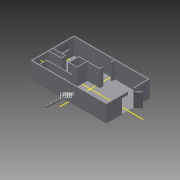
# Autodesk Inventor part: West_Structure_Hose_Test_2nd_Floor
Saved by Autodesk Inventor 2013 SP2 (Build 170200200, 200)
## iProperties
Created: 2013-07-10
Part Number: West_Structure_Hose_Test_2nd_Floor
Material: Generic
Document SubType Name: Modeling
Designer: jmw3
Density: 1 g/cm^3
Author: jmw3
Autodesk Inventor part; units mm, degrees
ref_plane "YZ Plane" through (0, 0, 0) normal (1, 0, 0) x (0, 1, 0)
ref_plane "XZ Plane" through (0, 0, 0) normal (0, 1, 0) x (-1, 0, 0)
ref_plane "XY Plane" through (0, 0, 0) normal (0, 0, 1) x (1, 0, 0)
sketch "Sketch1" plane through (0, 0, 0) normal (0, 0, 1) x (1, 0, 0)
  line L0 (-5588, 3200.4) -> (5588, 3200.4)
  line L1 (5588, -3200.4) -> (-5588, -3200.4)
  line L2 (-3958.3754, 3048) -> (-719.8754, 3048)
  line L3 (5435.6, 914.4) -> (5588, 914.4)
  line L4 (5588, -914.4) -> (5435.6, -914.4)
  line L5 (-4072.6754, 3048) -> (-605.5754, 3048)
  line L6 (5588, 3200.4) -> (5588, 914.4)
  line L7 (5588, -914.4) -> (5588, -3200.4)
  line L8 (5435.6, 3048) -> (5435.6, 914.4)
  line L9 (5435.6, -914.4) -> (5435.6, -3048)
  line L10 (-5588, 894.5564) -> (-5588, 3200.4)
  line L11 (-5435.6, 76.2) -> (-5435.6, 3048)
  line L12 (0, -4480.56) -> (0, 4480.56) projected
  line L13 (-7823.2, 0) -> (7823.2, 0) projected
  line L14 (-863.6, -3048) -> (-863.6, -2006.6)
  line L15 (-863.6, -2006.6) -> (-4381.5, -2006.6)
  line L16 (-4495.8, -2006.6) -> (-4495.8, -3048)
  line L17 (-5435.6, 76.2) -> (-3581.4, 76.2)
  line L18 (-3581.4, 76.2) -> (-3581.4, -685.8)
  line L19 (-3581.4, -685.8) -> (-5435.6, -685.8)
  line L20 (-5435.6, -571.5) -> (-5435.6, -38.1)
  line L21 (-5435.6, -38.1) -> (-3695.7, -38.1)
  line L22 (-3695.7, -38.1) -> (-3695.7, -571.5)
  line L23 (-3695.7, -571.5) -> (-5435.6, -571.5)
  line L24 (-5435.6, -571.5) -> (-5435.6, -38.1)
  line L25 (-5588, -965.2) -> (-5435.6, -965.2)
  line L26 (-5435.6, -1879.6) -> (-5588, -1879.6)
  line L27 (-5435.6, -3048) -> (-5435.6, -1879.6)
  line L28 (-5588, -3200.4) -> (-5588, -1879.6)
  line L29 (-5588, -965.2) -> (-5588, 914.4)
  line L30 (-2590.8, 914.4) -> (-1377.4097, 914.4)
  line L31 (-1244.6, 800.1) -> (-1244.6, -685.8)
  line L32 (-1244.6, -685.8) -> (-2590.8, -685.8)
  line L33 (-2590.8, -685.8) -> (-2590.8, 914.4)
  line L34 (-1377.4097, 914.4) -> (508, 914.4)
  line L35 (622.3, 952.5) -> (622.3, 800.1)
  line L36 (622.3, 800.1) -> (-1244.6, 800.1)
  line L37 (508, 914.4) -> (508, 1314.45)
  line L38 (508, 1314.45) -> (622.3, 1314.45)
  line L39 (622.3, 1314.45) -> (622.3, 800.1)
  line L40 (622.3, 3048) -> (622.3, 2533.65)
  line L41 (622.3, 2533.65) -> (508, 2533.65)
  line L42 (508, 2533.65) -> (508, 3048)
  line L43 (-2476.5, 800.1) -> (-1358.9, 800.1)
  line L44 (-1358.9, 800.1) -> (-1358.9, -571.5)
  line L45 (-1358.9, -571.5) -> (-2476.5, -571.5)
  line L46 (-2476.5, -571.5) -> (-2476.5, 800.1)
  line L47 (-749.3, -3048) -> (-749.3, -1892.3)
  line L48 (-749.3, -1892.3) -> (-4495.8, -1892.3)
  line L49 (-4495.8, -1892.3) -> (-4495.8, -2006.6)
  line L50 (-5435.6, 3048) -> (508, 3048)
  line L51 (622.3, 3048) -> (5435.6, 3048)
  line L52 (-4381.5, -2006.6) -> (-4381.5, -3048)
  line L53 (-863.6, -2006.6) -> (-1060.3581, -2006.6)
  line L54 (-5435.6, -965.2) -> (-5435.6, -685.8)
  line L55 (-5435.6, -571.5) -> (-5435.6, -38.1)
  line L56 (-4495.8, -3048) -> (-5435.6, -3048)
  line L57 (5435.6, -3048) -> (-749.3, -3048)
  line L58 (-863.6, -3048) -> (-4381.5, -3048)
  line L59 (880.3246, -3048) -> (-749.3, -3048)
  line L60 (-5435.6, -38.1) -> (-5435.6, -571.5)
  line L61 (-5435.6, -685.8) -> (-5435.6, -965.2)
  line L62 (-5435.6, -685.8) -> (-3581.4, -685.8)
  line L63 (-5435.6, 76.2) -> (-3581.4, 76.2)
  line L64 (-5435.6, 76.2) -> (-5435.6, 3048)
  line L65 (-5435.6, -685.8) -> (-5435.6, -965.2)
  line L66 (-5435.6, -965.2) -> (-5588, -965.2)
  line L67 (-5588, -965.2) -> (-5588, 3200.4)
  line L68 (-5435.6, 3048) -> (-5435.6, 76.2)
  line L69 (-5435.6, 76.2) -> (-3581.4, 76.2)
  line L70 (-3581.4, 76.2) -> (-3581.4, -685.8)
  line L71 (-3581.4, -685.8) -> (-5435.6, -685.8)
  line L72 (-5435.6, -571.5) -> (-3695.7, -571.5)
  line L73 (-3695.7, -571.5) -> (-3695.7, -38.1)
  line L74 (-3695.7, -38.1) -> (-5435.6, -38.1)
  line L75 (-5435.6, -38.1) -> (-5435.6, -571.5)
  dimension "d14" = 1828.8
  dimension "d90" = 6299.2
  dimension "d94" = 114.3
  dimension "d95" = 114.3
  dimension "d96" = 114.3
  dimension "d99" = 914.4
  dimension "d100" = 152.4
  dimension "d102" = 939.8
  dimension "d104" = 990.6
  dimension "d105" = 114.3
  dimension "d106" = 114.3
  dimension "d107" = 114.3
  dimension "d108" = 114.3
  dimension "d109" = 114.3
  dimension "d110" = 6680.2
  dimension "d112" = 1219.2
  dimension "d120" = 152.4
  dimension "d122" = 2971.8
  dimension "d123" = 2286
  dimension "d124" = 5943.6
  dimension "d125" = 114.3
  dimension "d127" = 114.3
  dimension "d128" = 6400.8
  dimension "d129" = 152.4
  dimension "d130" = 1168.4
  dimension "d131" = 1041.4
  dimension "d132" = 114.3
  dimension "d133" = 1854.2
  dimension "d134" = 2362.2
  dimension "d135" = 10871.2
  dimension "d236" = 2133.6
  dimension "d237" = 514.35
  dimension "d238" = 114.3
  constraints: 148 end point, 38 parallel, 28 perpendicular, 26 collinear, 12 horizontal, 3 point on line, 3 other
  measures "d14" distance between parallel lines of L4 L3
  measures "d90" distance between parallel lines of L9 L14
  measures "d94" distance between parallel lines of L19 L23
  measures "d95" distance between parallel lines of L18 L22
  measures "d96" distance between parallel lines of L17 L21
  measures "d99" distance between parallel lines of L25 L26
  measures "d100" distance between parallel lines of L10 L11
  measures "d102" distance between parallel lines of L27 L16
  measures "d104" distance between parallel lines of L18 L33
  measures "d105" distance between parallel lines of L33 L46
  measures "d106" distance between parallel lines of L31 L44
  measures "d107" distance between parallel lines of L32 L45
  measures "d108" distance between parallel lines of L30 L43
  measures "d109" distance between parallel lines of L39 L37
  measures "d110" distance between parallel lines of L8 L31
  measures "d112" distance from line of L38.end L41
  measures "d120" distance between parallel lines of L50 L0
  measures "d122" distance between parallel lines of L50 L17
  measures "d123" distance between parallel lines of L1 L4
  measures "d124" distance between parallel lines of L11 L37
  measures "d125" distance between parallel lines of L16 L52
  measures "d127" distance between parallel lines of L14 L47
  measures "d128" distance between parallel lines of L1 L0
  measures "d129" distance between parallel lines of L1 L57
  measures "d130" distance between parallel lines of L56 L26
  measures "d131" distance between parallel lines of L58 L15
  measures "d132" distance between parallel lines of L15 L48
  measures "d133" distance between parallel lines of L54 L18
  measures "d134" distance between parallel lines of L56 L19
  measures "d135" distance between parallel lines of L9 L27
  measures "d236" distance between parallel lines of L50 L30
  measures "d237" distance between parallel lines of L36 L38
  measures "d238" distance of L40.end L41.end
extrude "Extrusion7" add sketch "Sketch1" along normal blind 2463.8 contours L57 L9 L4 L7 L1 L12 | L12 L1 L28 L26 L27 L56 L16 L49 L48 L47 L57 | L0 L12 L50 L5 L2 L11 L17 L18 L13 L29 L10 | L0 L6 L3 L8 L51 L40 L41 L42 L50 L12 | L34 L37 L38 L39 L35 L36 L12 | L12 L36 L31 L13 L44 L43 L46 L33 L30 L34 | L13 L18 L19 L54 L25 L29 | L13 L46 L45 L44 L31 L32 L33
sketch "Sketch4" plane through (0, 0, 0) normal (0, 0, -1) x (-1, 0, 0)
  line L0 (4381.5, -3048) -> (863.6, -3048) projected
  line L1 (863.6, -3048) -> (863.6, -2006.6) projected
  line L2 (863.6, -2006.6) -> (4381.5, -2006.6) projected
  line L3 (4381.5, -2006.6) -> (4381.5, -3048) projected
  line L4 (-5435.6, -3048) -> (749.3, -3048) projected
  line L5 (-5435.6, -914.4) -> (-5435.6, -3048) projected
  line L6 (-5588, -914.4) -> (-5435.6, -914.4) projected
  line L7 (-5588, -3200.4) -> (-5588, -914.4) projected
  line L8 (5588, -3200.4) -> (-5588, -3200.4) projected
  line L9 (5588, -1879.6) -> (5588, -3200.4) projected
  line L10 (5435.6, -1879.6) -> (5588, -1879.6) projected
  line L11 (5435.6, -3048) -> (5435.6, -1879.6) projected
  line L12 (4495.8, -3048) -> (5435.6, -3048) projected
  line L13 (4495.8, -1892.3) -> (4495.8, -3048) projected
  line L14 (749.3, -1892.3) -> (4495.8, -1892.3) projected
  line L15 (749.3, -3048) -> (749.3, -1892.3) projected
  line L16 (3695.7, -571.5) -> (3695.7, -38.1) projected
  line L17 (3695.7, -38.1) -> (5435.6, -38.1) projected
  line L18 (5435.6, -38.1) -> (5435.6, -571.5) projected
  line L19 (5435.6, -571.5) -> (3695.7, -571.5) projected
  line L20 (5435.6, 3048) -> (-508, 3048) projected
  line L21 (5435.6, 76.2) -> (5435.6, 3048) projected
  line L22 (3581.4, 76.2) -> (5435.6, 76.2) projected
  line L23 (3581.4, -685.8) -> (3581.4, 76.2) projected
  line L24 (5435.6, -685.8) -> (3581.4, -685.8) projected
  line L25 (5435.6, -965.2) -> (5435.6, -685.8) projected
  line L26 (5588, -965.2) -> (5435.6, -965.2) projected
  line L27 (5588, 3200.4) -> (5588, -965.2) projected
  line L28 (-5588, 3200.4) -> (5588, 3200.4) projected
  line L29 (-5588, 914.4) -> (-5588, 3200.4) projected
  line L30 (-5435.6, 914.4) -> (-5588, 914.4) projected
  line L31 (-5435.6, 3048) -> (-5435.6, 914.4) projected
  line L32 (-622.3, 3048) -> (-5435.6, 3048) projected
  line L33 (-622.3, 2533.65) -> (-622.3, 3048) projected
  line L34 (-508, 2533.65) -> (-622.3, 2533.65) projected
  line L35 (-508, 3048) -> (-508, 2533.65) projected
  line L36 (1358.9, -571.5) -> (1358.9, 800.1) projected
  line L37 (1358.9, 800.1) -> (2476.5, 800.1) projected
  line L38 (2476.5, 800.1) -> (2476.5, -571.5) projected
  line L39 (2476.5, -571.5) -> (1358.9, -571.5) projected
  line L40 (2590.8, 914.4) -> (-508, 914.4) projected
  line L41 (-508, 914.4) -> (-508, 1314.45) projected
  line L42 (-508, 1314.45) -> (-622.3, 1314.45) projected
  line L43 (-622.3, 1314.45) -> (-622.3, 800.1) projected
  line L44 (-622.3, 800.1) -> (1244.6, 800.1) projected
  line L45 (1244.6, 800.1) -> (1244.6, -685.8) projected
  line L46 (1244.6, -685.8) -> (2590.8, -685.8) projected
  line L47 (2590.8, -685.8) -> (2590.8, 914.4) projected
  line L48 (-5588, 3200.4) -> (5588, 3200.4)
  line L49 (5588, 3200.4) -> (5588, -2006.6)
  line L50 (5588, -2006.6) -> (-5588, -2006.6)
  line L51 (-5588, -2006.6) -> (-5588, 3200.4)
  line L52 (-5588, -2006.6) -> (863.6, -2006.6)
  line L53 (863.6, -2006.6) -> (863.6, -3200.4)
  line L54 (863.6, -3200.4) -> (-5588, -3200.4)
  line L55 (-5588, -3200.4) -> (-5588, -2006.6)
  line L56 (4381.5, -2006.6) -> (5588, -2006.6)
  line L57 (5588, -2006.6) -> (5588, -3200.4)
  line L58 (5588, -3200.4) -> (4381.5, -3200.4)
  line L59 (4381.5, -3200.4) -> (4381.5, -2006.6)
  line L60 (4381.5, -3048) -> (863.6, -3048)
  line L61 (863.6, -3048) -> (863.6, -3200.4)
  line L62 (863.6, -3200.4) -> (4381.5, -3200.4)
  line L63 (4381.5, -3200.4) -> (4381.5, -3048)
  line L64 (863.6, -3200.4) -> (4381.5, -3200.4)
  line L65 (4381.5, -3200.4) -> (4381.5, -2895.6)
  line L66 (4381.5, -2895.6) -> (863.6, -2895.6)
  line L67 (863.6, -2895.6) -> (863.6, -3200.4)
  point P0 (0, 0)
  dimension "d192" = 889
  constraints: 40 end point, 10 parallel, 5 horizontal, 5 perpendicular, 3 point on line
  measures "d192" distance between parallel lines of L66 L2
extrude "Extrusion8" add sketch "Sketch4" against normal blind 25.4 contours L59 L8 L53 L0 | L3 L50 L13 L12 L11 L9 L8 L59 | L53 L8 L7 L50 L5 L4 L15 L1 | L2 L50 L15 L14 L13 | L50 L11 L12 L13 | L13 L14 L15 L50 L5 L6 L51 L30 L31 L32 L33 L34 L35 L20 L21 L22 L23 L24 L25 L26 L49 L10 L11 | L50 L11 L10 L9 | L15 L4 L5 L50 | L7 L6 L5 L50 | L26 L25 L24 L23 L22 L21 L20 L35 L34 L33 L32 L31 L30 L29 L28 L27 | L16 L17 L18 L19 | L36 L37 L38 L39 | L47 L46 L45 L44 L43 L42 L41 L40
sketch "Sketch5" plane through (-749.3, -3048, 2463.8) normal (1, 0, 0) x (0, 0, -1)
  line L0 (2438.4, 0) -> (2438.4, 1155.7) projected
  line L1 (2438.4, 1155.7) -> (0, 1155.7) projected
  line L2 (2438.4, 114.3) -> (406.4, 114.3)
  line L3 (406.4, 114.3) -> (406.4, 927.1)
  line L4 (406.4, 927.1) -> (2438.4, 927.1)
  line L5 (2438.4, 927.1) -> (2438.4, 114.3)
  line L6 (2438.4, 165.1) -> (457.2, 165.1)
  line L7 (457.2, 165.1) -> (457.2, 876.3)
  line L8 (457.2, 876.3) -> (2438.4, 876.3)
  line L9 (2438.4, 876.3) -> (2438.4, 165.1)
  point P0 (2463.8, 3048)
  dimension "d140" = 2032
  dimension "d142" = 228.6
  dimension "d143" = 812.8
  dimension "d144" = 1981.2
  dimension "d145" = 711.2
  dimension "d146" = 50.8
  constraints: 16 end point, 4 parallel, 2 horizontal, 2 perpendicular, 2 point on line
  measures "d140" distance between parallel lines of L5 L3
  measures "d142" distance between parallel lines of L1 L4
  measures "d143" distance between parallel lines of L4 L2
  measures "d144" distance between parallel lines of L9 L7
  measures "d145" distance between parallel lines of L6 L8
  measures "d146" distance between parallel lines of L2 L6
extrude "Extrusion9" cut sketch "Sketch5" against normal blind 50.8 contours L2 L3 L4 L0 L8 L7 L6
extrude "Extrusion10" cut sketch "Sketch5" against normal up to surface (114.3 mm away) contours L6 L7 L8 L0
sketch "Sketch6" plane through (0, 0, 2463.8) normal (0, 0, 1) x (1, 0, 0)
  line L0 (-3695.7, -38.1) -> (-3695.7, -571.5) projected
  line L1 (-3695.7, -571.5) -> (-5435.6, -571.5) projected
  line L2 (-5435.6, -571.5) -> (-5435.6, -38.1) projected
  line L3 (-5435.6, -38.1) -> (-3695.7, -38.1) projected
  line L4 (-5435.6, 3048) -> (508, 3048) projected
  line L5 (508, 3048) -> (508, 2533.65) projected
  line L6 (508, 2533.65) -> (622.3, 2533.65) projected
  line L7 (622.3, 2533.65) -> (622.3, 3048) projected
  line L8 (622.3, 3048) -> (5435.6, 3048) projected
  line L9 (5435.6, 3048) -> (5435.6, 914.4) projected
  line L10 (5435.6, 914.4) -> (5588, 914.4) projected
  line L11 (5588, 914.4) -> (5588, 3200.4) projected
  line L12 (5588, 3200.4) -> (-5588, 3200.4) projected
  line L13 (-5588, 3200.4) -> (-5588, -965.2) projected
  line L14 (-5588, -965.2) -> (-5435.6, -965.2) projected
  line L15 (-5435.6, -965.2) -> (-5435.6, -685.8) projected
  line L16 (-5435.6, -685.8) -> (-3581.4, -685.8) projected
  line L17 (-3581.4, -685.8) -> (-3581.4, 76.2) projected
  line L18 (-3581.4, 76.2) -> (-5435.6, 76.2) projected
  line L19 (-5435.6, 76.2) -> (-5435.6, 3048) projected
  line L20 (-1358.9, 800.1) -> (-1358.9, -571.5) projected
  line L21 (-1358.9, -571.5) -> (-2476.5, -571.5) projected
  line L22 (-2476.5, -571.5) -> (-2476.5, 800.1) projected
  line L23 (-2476.5, 800.1) -> (-1358.9, 800.1) projected
  line L24 (508, 914.4) -> (-2590.8, 914.4) projected
  line L25 (-2590.8, 914.4) -> (-2590.8, -685.8) projected
  line L26 (-2590.8, -685.8) -> (-1244.6, -685.8) projected
  line L27 (-1244.6, -685.8) -> (-1244.6, 800.1) projected
  line L28 (-1244.6, 800.1) -> (622.3, 800.1) projected
  line L29 (622.3, 800.1) -> (622.3, 1314.45) projected
  line L30 (622.3, 1314.45) -> (508, 1314.45) projected
  line L31 (508, 1314.45) -> (508, 914.4) projected
  line L32 (5435.6, 914.4) -> (5588, 914.4)
  line L33 (5588, 914.4) -> (5588, -914.4)
  line L34 (5588, -914.4) -> (5435.6, -914.4)
  line L35 (5435.6, -914.4) -> (5435.6, 914.4)
  line L36 (-5588, -965.2) -> (-5435.6, -965.2)
  line L37 (-5435.6, -965.2) -> (-5435.6, -1879.6)
  line L38 (-5435.6, -1879.6) -> (-5588, -1879.6)
  line L39 (-5588, -1879.6) -> (-5588, -965.2)
  point P0 (0, 0)
  constraints: 16 end point, 4 parallel, 2 horizontal, 2 perpendicular
extrude "Extrusion11" add sketch "Sketch6" against normal blind 406.4 contours L37 L38 L39 L14 | L10 L33 L34 L35
sketch "Sketch7" plane through (-5435.6, 76.2, 2463.8) normal (1, 0, 0) x (0, 0, -1)
  line L0 (2438.4, 0) -> (2438.4, 2971.8) projected
  line L1 (2438.4, 2971.8) -> (0, 2971.8) projected
  line L2 (431.8, 647.7) -> (1346.2, 647.7)
  line L3 (1346.2, 647.7) -> (1346.2, 2324.1)
  line L4 (1346.2, 2324.1) -> (431.8, 2324.1)
  line L5 (431.8, 2324.1) -> (431.8, 647.7)
  point P0 (2463.8, -76.2)
  dimension "d153" = 1676.4
  dimension "d155" = 914.4
  dimension "d156" = 1092.2
  dimension "d157" = 647.7
  constraints: 8 end point, 2 parallel, 1 horizontal, 1 perpendicular
  measures "d153" distance between parallel lines of L2 L4
  measures "d155" distance between parallel lines of L5 L3
  measures "d156" distance between parallel lines of L0 L3
  measures "d157" distance between parallel lines of L1 L4
extrude "Extrusion12" cut sketch "Sketch7" against normal up to surface (152.4 mm away)
sketch "Sketch9" plane through (-863.6, -3048, 2463.8) normal (-1, 0, 0) x (0, 0, 1)
  line L0 (-2463.8, 0) -> (-2438.4, 0)
  line L1 (-2438.4, 0) -> (-2438.4, 152.4)
  line L2 (-2438.4, 152.4) -> (-2463.8, 152.4)
  line L3 (-2463.8, 152.4) -> (-2463.8, 0)
  point P0 (-2463.8, 3048)
  dimension "d193" = 152.4
  constraints: 8 end point, 2 parallel, 1 horizontal, 1 perpendicular
  measures "d193" distance between parallel lines of L2 L0
extrude "Extrusion14" add sketch "Sketch9" along normal up to surface (3517.9 mm away)
sketch "Sketch11" plane through (0, 0, 2057.4) normal (0, 0, -1) x (-1, 0, 0)
  line L0 (-5435.6, -914.4) -> (-5435.6, 914.4) projected
  line L1 (-5588, 914.4) -> (-5588, -914.4) projected
  line L2 (7823.2, 0) -> (-7823.2, 0) projected
  line L3 (-5588, 12.7) -> (-5435.6, 12.7)
  line L4 (-5435.6, 12.7) -> (-5435.6, -12.7)
  line L5 (-5435.6, -12.7) -> (-5588, -12.7)
  line L6 (-5588, -12.7) -> (-5588, 12.7)
  point P0 (0, 0)
  dimension "d230" = 25.4
  constraints: 8 end point, 2 parallel, 2 point on line, 1 horizontal, 1 perpendicular, 1 other
  measures "d230" distance between parallel lines of L5 L3
extrude "Extrusion16" add sketch "Sketch11" along normal blind 25.4
sketch "Sketch10" plane through (-4381.5, -2006.6, 2463.8) normal (0, -1, 0) x (1, 0, 0)
  line L0 (3517.9, -2463.8) -> (3517.9, 0) projected
  line L1 (0, 0) -> (3517.9, 0) projected
  line L2 (3632.2, -2438.4) -> (-114.3, -2438.4) projected
  line L3 (-114.3, -2438.4) -> (-114.3, 0) projected
  line L4 (3632.2, 0) -> (-114.3, 0) projected
  line L5 (3632.2, -2438.4) -> (3632.2, 0) projected
  line L6 (850.9, -5016.5) -> (1041.4, -5016.5)
  line L7 (1041.4, -5016.5) -> (1041.4, -4832.35)
  line L8 (1041.4, -4832.35) -> (914.4, -4832.35)
  line L9 (1041.4, -4832.35) -> (1231.9, -4832.35)
  line L10 (1231.9, -4832.35) -> (1231.9, -4648.2)
  line L11 (1231.9, -4648.2) -> (1041.4, -4648.2)
  line L12 (1041.4, -4648.2) -> (1041.4, -4832.35)
  line L13 (1612.9, -4464.05) -> (1612.9, -4279.9)
  line L14 (1422.4, -4648.2) -> (1422.4, -4464.05)
  line L15 (1422.4, -4464.05) -> (1612.9, -4464.05)
  line L16 (1612.9, -4279.9) -> (1422.4, -4279.9)
  line L17 (1422.4, -4279.9) -> (1422.4, -4464.05)
  line L18 (1231.9, -4648.2) -> (1422.4, -4648.2)
  line L19 (1422.4, -4464.05) -> (1231.9, -4464.05)
  line L20 (1231.9, -4464.05) -> (1231.9, -4648.2)
  line L21 (2184.4, -3911.6) -> (2184.4, -3727.45)
  line L22 (2184.4, -3543.3) -> (2184.4, -3727.45)
  line L23 (2184.4, -3727.45) -> (2374.9, -3727.45)
  line L24 (2374.9, -3543.3) -> (2184.4, -3543.3)
  line L25 (1993.9, -3727.45) -> (1993.9, -3911.6)
  line L26 (1993.9, -3911.6) -> (2184.4, -3911.6)
  line L27 (2184.4, -3727.45) -> (1993.9, -3727.45)
  line L28 (2374.9, -3727.45) -> (2374.9, -3543.3)
  line L29 (1993.9, -4095.75) -> (1993.9, -3911.6)
  line L30 (1993.9, -3911.6) -> (1803.4, -3911.6)
  line L31 (1803.4, -4095.75) -> (1993.9, -4095.75)
  line L32 (1803.4, -3911.6) -> (1803.4, -4095.75)
  line L33 (1803.4, -4279.9) -> (1803.4, -4095.75)
  line L34 (1803.4, -4095.75) -> (1612.9, -4095.75)
  line L35 (1612.9, -4279.9) -> (1803.4, -4279.9)
  line L36 (1612.9, -4095.75) -> (1612.9, -4279.9)
  line L37 (2755.9, -3175) -> (2946.4, -3175)
  line L38 (2946.4, -3175) -> (2946.4, -2990.85)
  line L39 (2946.4, -2806.7) -> (2946.4, -2990.85)
  line L40 (2946.4, -2990.85) -> (3136.9, -2990.85)
  line L41 (3136.9, -2806.7) -> (2946.4, -2806.7)
  line L42 (3136.9, -2990.85) -> (3136.9, -2806.7)
  line L43 (3136.9, -2622.55) -> (3136.9, -2806.7)
  line L44 (3136.9, -2806.7) -> (3327.4, -2806.7)
  line L45 (3327.4, -2622.55) -> (3136.9, -2622.55)
  line L46 (3327.4, -2806.7) -> (3327.4, -2622.55)
  line L47 (2374.9, -3359.15) -> (2374.9, -3543.3)
  line L48 (2374.9, -3543.3) -> (2565.4, -3543.3)
  line L49 (2565.4, -3543.3) -> (2565.4, -3359.15)
  line L50 (2565.4, -3359.15) -> (2374.9, -3359.15)
  line L51 (2565.4, -3175) -> (2565.4, -3359.15)
  line L52 (2565.4, -3359.15) -> (2755.9, -3359.15)
  line L53 (2755.9, -3175) -> (2565.4, -3175)
  line L54 (2755.9, -3359.15) -> (2755.9, -3175)
  line L55 (2755.9, -2990.85) -> (2755.9, -3175)
  line L56 (2946.4, -2990.85) -> (2755.9, -2990.85)
  line L57 (3327.4, -2622.55) -> (3517.9, -2622.55)
  line L58 (3517.9, -2622.55) -> (3517.9, -2438.4)
  line L59 (3517.9, -2438.4) -> (3327.4, -2438.4)
  line L60 (3327.4, -2438.4) -> (3327.4, -2622.55)
  line L61 (3136.9, -2762.25) -> (3327.4, -2762.25)
  line L62 (1041.4, -4832.35) -> (850.9, -4832.35)
  line L63 (850.9, -4832.35) -> (850.9, -5016.5)
  line L64 (1041.4, -5016.5) -> (1041.4, -4832.35)
  line L65 (850.9, -5016.5) -> (660.4, -5016.5)
  line L66 (660.4, -5016.5) -> (660.4, -5200.65)
  line L67 (660.4, -5200.65) -> (850.9, -5200.65)
  line L68 (850.9, -5200.65) -> (850.9, -5016.5)
  point P0 (4381.5, -2463.8)
  dimension "d197" = 184.15
  dimension "d198" = 190.5
  dimension "d199" = 184.15
  dimension "d200" = 190.5
  dimension "d201" = 184.15
  dimension "d202" = 190.5
  dimension "d203" = 184.15
  dimension "d204" = 190.5
  dimension "d205" = 184.15
  dimension "d206" = 190.5
  dimension "d207" = 184.15
  dimension "d208" = 190.5
  dimension "d209" = 184.15
  dimension "d210" = 190.5
  dimension "d211" = 184.15
  dimension "d212" = 190.5
  dimension "d213" = 184.15
  dimension "d214" = 190.5
  dimension "d215" = 184.15
  dimension "d216" = 190.5
  dimension "d217" = 184.15
  dimension "d218" = 190.5
  dimension "d219" = 184.15
  dimension "d220" = 190.5
  dimension "d221" = 184.15
  dimension "d222" = 184.15
  dimension "d223" = 190.5
  dimension "d224" = 190.5
  dimension "d225" = 190.5
  dimension "d226" = 184.15
  constraints: 127 end point, 31 parallel, 16 horizontal, 16 perpendicular, 14 collinear, 2 point on line
  measures "d197" distance between parallel lines of L8 L6
  measures "d198" distance between parallel lines of L10 L12
  measures "d199" distance between parallel lines of L11 L9
  measures "d200" distance between parallel lines of L20 L14
  measures "d201" distance between parallel lines of L19 L18
  measures "d202" distance between parallel lines of L13 L17
  measures "d203" distance between parallel lines of L16 L15
  measures "d204" distance between parallel lines of L36 L33
  measures "d205" distance between parallel lines of L34 L35
  measures "d206" distance between parallel lines of L29 L32
  measures "d207" distance between parallel lines of L30 L31
  measures "d208" distance between parallel lines of L25 L21
  measures "d209" distance between parallel lines of L27 L26
  measures "d210" distance between parallel lines of L28 L22
  measures "d211" distance between parallel lines of L24 L23
  measures "d212" distance between parallel lines of L49 L47
  measures "d213" distance between parallel lines of L50 L48
  measures "d214" distance between parallel lines of L51 L54
  measures "d215" distance between parallel lines of L53 L52
  measures "d216" distance between parallel lines of L38 L55
  measures "d217" distance between parallel lines of L56 L37
  measures "d218" distance between parallel lines of L39 L42
  measures "d219" distance between parallel lines of L41 L40
  measures "d220" distance between parallel lines of L46 L43
  measures "d221" distance between parallel lines of L45 L44
  measures "d222" distance between parallel lines of L57 L59
  measures "d223" distance between parallel lines of L60 L58
  measures "d224" distance between parallel lines of L63 L64
  measures "d225" distance between parallel lines of L68 L66
  measures "d226" distance between parallel lines of L65 L67
extrude "Extrusion15" add sketch "Sketch10" along normal blind 889 contours L58 L57 L60 L2 L0 | L68 L67 L66 L65 | L7 L6 L63 L62 L8 | L10 L9 L12 L11 | L14 L18 L20 L19 | L13 L15 L17 L16 | L33 L35 L36 L34 | L29 L31 L32 L30 | L21 L26 L25 L27 | L28 L23 L22 L24 | L49 L48 L47 L50 | L54 L52 L51 L53 | L38 L37 L55 L56 | L42 L40 L39 L41 | L46 L61 L43 L45
sketch "Sketch12" plane through (0, 0, 25.4) normal (0, 0, 1) x (1, 0, 0)
  line L0 (-1054.1, -2895.6) -> (-863.6, -2895.6)
  line L1 (-863.6, -2895.6) -> (-863.6, -2006.6)
  line L2 (-863.6, -2006.6) -> (-1054.1, -2006.6)
  line L3 (-1054.1, -2006.6) -> (-1054.1, -2895.6)
  point P0 (0, 0)
  constraints: 8 end point, 2 parallel, 1 horizontal, 1 perpendicular
extrude "Extrusion17" cut sketch "Sketch12" against normal blind 0.0254
sketch "Sketch13" plane through (0, 0, 25.4) normal (0, 0, 1) x (1, 0, 0)
  line L0 (-863.6, -2171.7) -> (-863.6, -2882.9) projected
  line L1 (5435.6, -3048) -> (-749.3, -3048) projected
  line L2 (-749.3, -2120.9) -> (-749.3, -1892.3) projected
  line L3 (-647.7, -2743.2) -> (-1079.5, -2743.2)
  line L4 (-1079.5, -2743.2) -> (-1079.5, -2311.4)
  line L5 (-7899.4, 0) -> (7835.9, 0) projected
  line L6 (0, -4480.56) -> (0, 4480.56) projected
  line L7 (-1079.5, -2311.4) -> (-647.7, -2743.2)
  line L8 (-5588, 723.9) -> (-5588, 2400.3) projected
  line L9 (-5435.6, 723.9) -> (-5588, 723.9) projected
  line L10 (-5435.6, 2400.3) -> (-5435.6, 723.9) projected
  line L11 (-5435.6, 2400.3) -> (-5588, 2400.3) projected
  line L12 (-687.6236, -2832.1) -> (-1039.5764, -2832.1)
  point P0 (0, 0)
  point P1 (-5588, 1841.5)
  point P2 (-5588, 1282.7)
  point P3 (-863.6, -2527.3)
  point P4 (-863.6, -2222.5)
  dimension "d252" = 431.8
  dimension "d253" = 431.8
  dimension "d256" = 215.9
  constraints: 8 end point, 3 parallel, 3 point on line, 2 other
  measures "d252" distance of L3.start L3.end
  measures "d253" distance of L3.end L4.end
  measures "d256" distance between parallel lines of L0 L4
extrude "Extrusion23" add sketch "Sketch13" along normal blind 25.4 contours L7 L3 L0 | L0 L3 L4 L7
sketch "Sketch16" plane through (0, 0, 2463.8) normal (0, 0, 1) x (1, 0, 0)
  line L0 (-863.6, -2006.6) -> (-863.6, -3048) projected
  line L1 (-800.1, -2171.7) -> (-800.1, -2882.9) projected
  line L2 (-800.1, -2882.9) -> (-863.6, -2882.9) projected
  line L3 (-863.6, -2171.7) -> (-863.6, -2882.9) projected
  line L4 (-800.1, -2171.7) -> (-863.6, -2171.7) projected
  line L5 (5588, 12.7) -> (5435.6, 12.7) projected
  line L6 (5435.6, 12.7) -> (5435.6, 914.4) projected
  line L7 (5588, 914.4) -> (5435.6, 914.4) projected
  line L8 (5588, 914.4) -> (5588, 12.7) projected
  line L9 (-749.3, -2933.7) -> (-749.3, -2120.9) projected
  line L10 (-749.3, -2933.7) -> (-800.1, -2933.7) projected
  line L11 (-800.1, -2933.7) -> (-800.1, -2120.9) projected
  line L12 (-749.3, -2120.9) -> (-800.1, -2120.9) projected
  line L13 (-749.3, -2120.9) -> (-863.6, -2120.9)
  line L14 (-863.6, -2120.9) -> (-863.6, -2933.7)
  line L15 (-863.6, -2933.7) -> (-749.3, -2933.7)
  line L16 (-749.3, -2933.7) -> (-749.3, -2120.9)
  line L17 (5435.6, -12.7) -> (5588, -12.7) projected
  line L18 (5435.6, 3048) -> (5435.6, -3048) projected
  line L19 (5588, -3200.4) -> (5588, 3200.4) projected
  line L20 (5435.6, 0) -> (5588, 0)
  line L21 (5588, 0) -> (5588, 914.4)
  line L22 (5588, 914.4) -> (5435.6, 914.4)
  line L23 (5435.6, 914.4) -> (5435.6, 0)
  point P0 (0, 0)
  constraints: 16 end point, 4 parallel, 2 horizontal, 2 perpendicular, 1 midpoint, 1 point on line
extrude "Extrusion24" cut sketch "Sketch16" against normal up to surface (2438.4 mm away) contours L13 L11 L4 L0 | L4 L1 L2 L0 | L12 L9 L10 L11 L1 | L2 L11 L15 L0 | L5 L6 L7 L8
extrude "Extrusion25" add sketch "Sketch13" along normal blind 25.4 contours L7 L3 L0 | L0 L3 L4 L7
sketch "Sketch17" plane through (0, 0, 2032) normal (0, 0, -1) x (-1, 0, 0)
  line L0 (-5435.6, -12.7) -> (-5435.6, 12.7) projected
  line L1 (-5435.6, 12.7) -> (-5588, 12.7) projected
  line L2 (-5588, 12.7) -> (-5588, -12.7) projected
  line L3 (-5588, -12.7) -> (-5435.6, -12.7) projected
  point P0 (0, 0)
extrude "Extrusion26" cut sketch "Sketch17" against normal up to surface (25.4 mm away)
sketch "Sketch18" plane through (5435.6, 12.7, 2057.4) normal (0, 1, 0) x (1, 0, 0)
  line L0 (152.4, 0) -> (0, 0) projected
  line L1 (0, -406.4) -> (0, 0) projected
  line L2 (152.4, -406.4) -> (0, -406.4) projected
  line L3 (152.4, 0) -> (152.4, -406.4) projected
  point P0 (-5435.6, 2057.4)
extrude "Extrusion27" cut sketch "Sketch18" against normal blind 12.7
sketch "Sketch19" plane through (0, 0, 25.4) normal (0, 0, 1) x (1, 0, 0)
  line L0 (5435.6, -3048) -> (-749.3, -3048) projected
  line L1 (-749.3, -2933.7) -> (55.4232, -3048)
  line L2 (55.4232, -3048) -> (71.4966, -2934.8358)
  line L3 (71.4966, -2934.8358) -> (-733.2266, -2820.5358)
  line L4 (-733.2266, -2820.5358) -> (-749.3, -2933.7)
  line L5 (5588, 914.4) -> (6276.6453, 1515.9771)
  line L6 (5588, 914.4) -> (5688.2628, 799.6258)
  line L7 (6276.6453, 1515.9771) -> (6376.9082, 1401.2028)
  line L8 (5688.2628, 799.6258) -> (6376.9082, 1401.2028)
  line L9 (-7899.4, 0) -> (7835.9, 0) projected
  point P0 (0, 0)
  dimension "d344" = 812.8
  dimension "d346" = 114.3
  dimension "d347" = 152.4
  dimension "d348" = 914.4
  constraints: 16 end point, 3 parallel, 3 perpendicular, 1 point on line
  measures "d344" distance between parallel lines of L2 L4
  measures "d346" distance between parallel lines of L1 L3
  measures "d347" distance between parallel lines of L8 L5
  measures "d348" distance between parallel lines of L6 L7
extrude "Extrusion28" add sketch "Sketch19" along normal blind 2032
sketch "Sketch20" plane through (0, 0, 50.8) normal (0, 0, 1) x (1, 0, 0)
  line L0 (-1079.5, -2743.2) -> (-647.7, -2743.2) projected
  line L1 (-647.7, -2743.2) -> (-1079.5, -2311.4) projected
  line L2 (-1079.5, -2311.4) -> (-1079.5, -2743.2) projected
  point P0 (0, 0)
  dimension "d318" = 304.8
  dimension "d319" = 431.8
  dimension "d320" = 431.8
  dimension "d321" = 215.9
  dimension "d322" = 304.8
  dimension "d323" = 431.8
  dimension "d324" = 431.8
  dimension "d325" = 215.9
  dimension "d326" = 558.8
  dimension "d327" = 558.8
extrude "Extrusion29" cut sketch "Sketch20" against normal up to surface (25.4 mm away)
body "Solid2"
